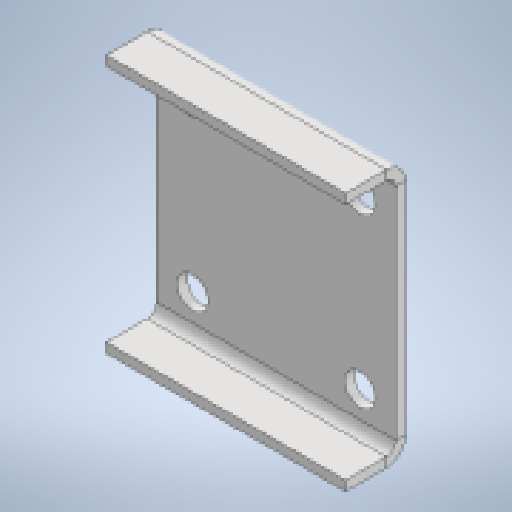
# Autodesk Inventor part: GBK-RK-0820 ring plate_CPY
Saved by Autodesk Inventor 2026.2 (Build 302298000, 298)
## iProperties
Created: 2024-05-23
Part Number: GBK-RK-0820 ring plate_CPY
Material: Generic
Document SubType Name: Sheet Metal
Designer: admin
Mass: 0.559799 g
Surface Area: 23.3947 cm^2
Volume: 0.559799 cm^3
Density: 1 g/cm^3
Flat Pattern Width: 14.4096 cm
Flat Pattern Length: 10 cm
Flat Pattern Area: 144.096 cm^2
Sheet Metal Rule: Default_mm
Sheet Metal Width: 144,096 mm
Sheet Metal Length: 100,000 mm
Sheet Metal Area: 14409,557 mm^2
Appearance: Default
Author: admin
Autodesk Inventor part; units mm, degrees
ref_plane "YZ Plane" through (0, 0, 0) normal (1, 0, 0) x (0, 1, 0)
ref_plane "XZ Plane" through (0, 0, 0) normal (0, 1, 0) x (-1, 0, 0)
ref_plane "XY Plane" through (0, 0, 0) normal (0, 0, 1) x (1, 0, 0)
sketch "Sketch1" plane through (0, 0, 0) normal (0, 0, 1) x (1, 0, 0)
  line L0 (-50, 50) -> (50, 50)
  line L1 (50, 50) -> (50, -50)
  line L2 (50, -50) -> (-50, -50)
  line L3 (-50, -50) -> (-50, 50)
  line L4 (-50, 50) -> (50, -50) construction
  line L5 (50, 50) -> (-50, -50) construction
  line L6 (0, 50) -> (0, -50) construction
  circle A0 centre (-35, -35) radius 6.5
  circle A1 centre (-35, 35) radius 6.5
  circle A2 centre (35, -35) radius 6.5
  circle A3 centre (35, 35) radius 6.5
  line L7 (35, 35) -> (-35, 35) construction
  line L8 (-35, 35) -> (-35, -35) construction
  line L9 (-35, -35) -> (35, -35) construction
  line L10 (35, -35) -> (35, 35) construction
  line L11 (35, 35) -> (-35, -35) construction
  line L12 (-35, 35) -> (35, -35) construction
  point P0 (0, 0)
  dimension "d0" = 100
  dimension "d1" = 100
  dimension "d19" = 13
  dimension "d20" = 70
  measures "d0" distance of L1.end L2.end
  measures "d1" distance of L0.end L1.end
  measures "d19" diameter of A0
  measures "d20" distance of L8.end L9.end
extrude "Plate1" add sketch "Sketch1" along normal blind 4
sketch "Sketch3" plane through (50, -54, 0) normal (0, 1, 0) x (-1, 0, 0)
  line L0 (100, 0) -> (0, 0)
  line L1 (0, 0) -> (0, 25)
  line L2 (0, 25) -> (100, 25)
  line L3 (100, 25) -> (100, 0)
  constraints: 8 end point
edge flange "Flange1" height 25 angle 90 thickness 4 bend radius 4 thickness toward (0, 1, 0) relief tear relief width 4 relief depth 2 corner gap 4 corner form 0 edges at (0, -50, 4) (0, 50, 4) wall of the first edge with corners at (-50, -54, 0) (50, -54, 0) (50, -54, 25) (-50, -54, 25)
bend "Bend1"
corner "Corner1"
equation "\"d0\" = d1"
equation "\"d2\" = Thickness"
equation "\"d21\" = BendReliefWidth"
equation "\"d22\" = BendReliefDepth"
equation "\"d23\" = MinimumRemnant"
equation "\"d24\" = TransitionRadius"
equation "\"d27\" = BendRadius"
equation "\"d28\" = CornerReliefSize"
equation "\"d29\" = GapSize"
equation "\"d30\" = JacobiRadiusSize"
equation "\"BendRadius\" = Thickness"
equation "\"BendReliefWidth\" = Thickness"
equation "\"BendReliefDepth\" = 0.5 * Thickness"
equation "\"CornerReliefSize\" = 4 * Thickness"
equation "\"MinimumRemnant\" = 2 * Thickness"
equation "\"TransitionRadius\" = BendRadius"
equation "\"JacobiRadiusSize\" = BendRadius"
equation "\"GapSize\" = Thickness"
equation "\"Thickness\" = 4"
body "Solid1"
